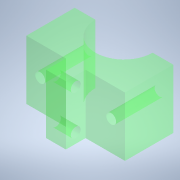
# Autodesk Inventor part: 3_Connettore_inf_INF
Saved by Autodesk Inventor 2020 (Build 240168000, 168)
## iProperties
Created: 2019-10-11
Part Number: 3_Connettore_inf_INF
Material: Generico
Document SubType Name: Modeling
Designer: socci
Density: 1 g/cm^3
Appearance: Verde
Author: socci
Autodesk Inventor part; units mm, degrees
ref_plane "YZ Plane" through (0, 0, 0) normal (1, 0, 0) x (0, 1, 0)
ref_plane "XZ Plane" through (0, 0, 0) normal (0, 1, 0) x (-1, 0, 0)
ref_plane "XY Plane" through (0, 0, 0) normal (0, 0, 1) x (1, 0, 0)
sketch "Schizzo1" plane through (0, 0, 0) normal (0, 0, 1) x (1, 0, 0)
  line L0 (-25, -15) -> (25, -15)
  line L1 (25, -15) -> (25, 15)
  line L2 (25, 15) -> (-25, 15)
  line L3 (-25, 15) -> (-25, -15)
  line L4 (-25, -15) -> (25, 15) construction
  line L5 (25, -15) -> (-25, 15) construction
  point P0 (0, 0)
  dimension "d0" = 50
  dimension "d1" = 30
  constraints: 12 end point, 2 midpoint, 2 parallel, 1 horizontal, 1 perpendicular
  measures "d0" distance of L2.end L1.end
  measures "d1" distance of L1.end L0.end
extrude "Estrusione1" add sketch "Schizzo1" against normal blind 24.5
sketch "Schizzo2" plane through (-25, 15, 0) normal (0, 1, 0) x (1, 0, 0)
  line L0 (50, 24.5) -> (0, 24.5) projected
  circle A0 centre (25, 24.5) radius 14.5
  point P0 (25, 0)
  dimension "d4" = 29
  constraints: 1 centre point, 1 midpoint
  measures "d4" diameter of A0
extrude "Estrusione2" cut sketch "Schizzo2" against normal blind 30
sketch "Schizzo3" plane through (0, 0, 0) normal (0, 0, 1) x (1, 0, 0)
  line L0 (25, 15) -> (-25, 15) projected
  line L1 (5, -15) -> (-5, -15)
  line L2 (-5, -15) -> (-5, 15)
  line L3 (-5, 15) -> (5, 15)
  line L4 (5, 15) -> (5, -15)
  line L5 (5, -15) -> (-5, 15) construction
  line L6 (-5, -15) -> (5, 15) construction
  point P0 (0, 0)
  dimension "d7" = 10
  constraints: 12 end point, 2 midpoint, 2 parallel, 1 horizontal, 1 perpendicular, 1 point on line
  measures "d7" distance of L2.end L3.end
extrude "Estrusione3" add sketch "Schizzo3" along normal blind 10
sketch "Schizzo4" plane through (0, 0, -24.5) normal (0, 0, -1) x (-1, 0, 0)
  circle A0 centre (-18, 0) radius 2.5 projected
  circle A1 centre (18, 0) radius 2.5 projected
  point P0 (0, 0)
hole "Foro1" at (18, 0, -24.5) at (-18, 0, -24.5) direction (0, 0, 1) diameter 5 end through all
sketch "Schizzo5" plane through (-5, -15, 0) normal (-1, 0, 0) x (0, 0, 1)
  line L0 (0, 0) -> (10, 0) projected
  line L1 (0, 0) -> (0, 30) projected
  line L2 (10, 0) -> (0, 0)
  line L3 (0, 0) -> (0, 10)
  line L4 (10, 10) -> (10, 0)
  line L5 (5, 0) -> (5, 5)
  line L6 (0, 30) -> (10, 30) projected
  line L7 (5, 30) -> (5, 25)
  point P0 (0, 15)
  dimension "d17" = 10
  dimension "d18" = 5
  dimension "d19" = 5
  constraints: 10 end point, 2 midpoint, 2 perpendicular, 1 horizontal, 1 parallel, 1 point on line, 1 vertical
  measures "d17" distance of L2.end L3.end
  measures "d18" distance of L5.start L5.end
  measures "d19" distance of L7.start L7.end
hole "Foro2" at (-5, 10, 5) at (-5, -10, 5) direction (1, 0, 0) diameter 5 end through all
